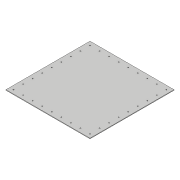
# Autodesk Inventor part: panel
Saved by Autodesk Inventor 2017 (Build 210142000, 142)
## iProperties
Created: 2016-07-20
Part Number: panel
Material: Generic
Document SubType Name: Modeling
Designer: Zuhra Abdurashidova
Density: 1 g/cm^3
Appearance: Default
Author: Zuhra Abdurashidova
Autodesk Inventor part; units mm, degrees
ref_plane "YZ Plane" through (0, 0, 0) normal (1, 0, 0) x (0, 1, 0)
ref_plane "XZ Plane" through (0, 0, 0) normal (0, 1, 0) x (-1, 0, 0)
ref_plane "XY Plane" through (0, 0, 0) normal (0, 0, 1) x (1, 0, 0)
sketch "Sketch1" plane through (0, 0, 0) normal (0, 1, 0) x (-1, 0, 0)
  line L0 (0, 0) -> (-440, 0)
  line L1 (-440, 0) -> (-440, -440)
  line L2 (-440, -440) -> (0, -440)
  line L3 (0, -440) -> (0, 0)
  dimension "d0" = 440
  dimension "d1" = 440
  constraints: 8 end point, 2 parallel, 1 horizontal, 1 perpendicular
  measures "d0" distance of L1.end L2.end
  measures "d1" distance of L0.end L1.end
extrude "panel body" add sketch "Sketch1" along normal blind 3
sketch "Sketch2" plane through (0, 3, 0) normal (0, 1, 0) x (1, 0, 0)
  line L0 (20, 20) -> (420, 20) construction
  line L1 (420, 20) -> (420, 420) construction
  line L2 (420, 420) -> (20, 420) construction
  line L3 (20, 420) -> (20, 20) construction
  line L4 (20, 20) -> (420, 420) construction
  line L5 (420, 20) -> (20, 420) construction
  line L6 (440, 440) -> (0, 440) projected
  line L7 (220, 440) -> (220, 3.9535) construction
  line L8 (0, 440) -> (0, 0) projected
  line L9 (0, 220) -> (440, 220) construction
  line L10 (440, 0) -> (440, 440) projected
  circle A0 centre (20, 420) radius 2.5
  circle A1 centre (70, 420) radius 2.5
  circle A2 centre (120, 420) radius 2.5
  circle A3 centre (170, 420) radius 2.5
  circle A4 centre (220, 420) radius 2.5
  circle A5 centre (270, 420) radius 2.5
  circle A6 centre (320, 420) radius 2.5
  circle A7 centre (370, 420) radius 2.5
  circle A8 centre (420, 420) radius 2.5
  circle A9 centre (420, 370) radius 2.5
  circle A10 centre (420, 320) radius 2.5
  circle A11 centre (420, 270) radius 2.5
  circle A12 centre (420, 220) radius 2.5
  circle A13 centre (420, 170) radius 2.5
  circle A14 centre (420, 120) radius 2.5
  circle A15 centre (420, 70) radius 2.5
  circle A16 centre (420, 20) radius 2.5
  circle A17 centre (370, 20) radius 2.5
  circle A18 centre (320, 20) radius 2.5
  circle A19 centre (270, 20) radius 2.5
  circle A20 centre (220, 20) radius 2.5
  circle A21 centre (170, 20) radius 2.5
  circle A22 centre (120, 20) radius 2.5
  circle A23 centre (70, 20) radius 2.5
  circle A24 centre (20, 20) radius 2.5
  circle A25 centre (20, 70) radius 2.5
  circle A26 centre (20, 120) radius 2.5
  circle A27 centre (20, 170) radius 2.5
  circle A28 centre (20, 220) radius 2.5
  circle A29 centre (20, 270) radius 2.5
  circle A30 centre (20, 320) radius 2.5
  circle A31 centre (20, 370) radius 2.5
  point P0 (220, 220)
  dimension "d161" = 400
  dimension "d162" = 400
  dimension "d163" = 5
  dimension "d210" = 50
  dimension "d217" = 50
  dimension "d224" = 50
  dimension "d231" = 50
  constraints: 32 centre point, 16 end point, 5 midpoint, 3 horizontal, 3 vertical, 2 parallel, 1 coincident, 1 perpendicular, 64 other
  measures "d161" distance of L2.end L1.end
  measures "d162" distance of L1.end L0.end
  measures "d163" diameter of A0
  measures "d210" distance of A0.centre A1.centre
  measures "d217" distance of A8.centre A9.centre
  measures "d224" distance of A16.centre A17.centre
  measures "d231" distance of A24.centre A25.centre
extrude "Extrusion4" cut sketch "Sketch2" against normal up to next
body "Solid3"
